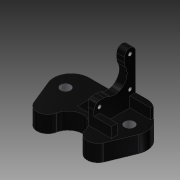
# Autodesk Inventor part: BackStopper
Saved by Autodesk Inventor 2015 (Build 190159000, 159)
## iProperties
Created: 2017-01-04
Part Number: BackStopper
Material: Generic
Document SubType Name: Modeling
Designer: Ernest
Density: 1 g/cm^3
Appearance: Default
Mass: 71.4554 g
Surface Area: 189.352 cm^2
Volume: 71.4554 cm^3
Author: Ernest
Autodesk Inventor part; units mm, degrees
ref_plane "YZ Plane" through (0, 0, 0) normal (1, 0, 0) x (0, 1, 0)
ref_plane "XZ Plane" through (0, 0, 0) normal (0, 1, 0) x (-1, 0, 0)
ref_plane "XY Plane" through (0, 0, 0) normal (0, 0, 1) x (1, 0, 0)
sketch "Sketch1" plane through (0, 0, 0) normal (0, 0, 1) x (1, 0, 0)
  circle A0 centre (0, 0) radius 8
  circle A1 centre (25.5147, 5) radius 3
  circle A2 centre (-25.5147, 5) radius 3
  circle A3 centre (32.5, 30) radius 5
  circle A4 centre (-32.5, 30) radius 5
  arc A5 (45.4578, 24.6994) -> (32.5, 44) centre (32.5, 30) ccw
  arc A6 (-32.5, 44) -> (-45.4578, 24.6994) centre (-32.5, 30) ccw
  line L0 (-24.3676, 0) -> (22.7562, 0) construction
  line L1 (-38.3266, 30) -> (45.5284, 30) construction
  line L2 (-33.7528, 8) -> (48.0284, 8) construction
  circle A7 centre (-25.5147, 5) radius 6
  circle A8 centre (25.5147, 5) radius 6
  arc A9 (14.72, 2.8846) -> (-15, 0) centre (0, 0) ccw
  arc A10 (-35.6958, 0.8353) -> (-14.72, 2.8846) centre (-25.5147, 5) ccw
  arc A11 (14.72, 2.8846) -> (35.6958, 0.8353) centre (25.5147, 5) ccw
  line L3 (-45.4578, 24.6994) -> (-35.6958, 0.8353)
  line L4 (35.6958, 0.8353) -> (45.4578, 24.6994)
  line L5 (-32.5, 44) -> (32.5, 44)
  dimension "d0" = 65
  dimension "d1" = 32.5
  dimension "d2" = 10
  dimension "d3" = 10
  dimension "d4" = 6
  dimension "d5" = 6
  dimension "d6" = 28
  dimension "d7" = 28
  dimension "d14" = 16
  dimension "d16" = 15
  dimension "d18" = 12
  dimension "d19" = 12
  dimension "d20" = 30
  dimension "d33" = 30
  dimension "d34" = 15
  constraints: 12 centre point, 12 end point, 11 point on circle, 10 tangent, 8 coincident, 4 horizontal, 4 point on line, 2 parallel
  measures "d0" distance of A3.centre A4.centre
  measures "d1" horizontal distance of point (0, 0) A4.centre
  measures "d2" diameter of A4
  measures "d3" diameter of A3
  measures "d4" diameter of A2
  measures "d5" diameter of A1
  measures "d6" diameter of A5
  measures "d7" diameter of A6
  measures "d14" diameter of A0
  measures "d18" diameter of A7
  measures "d19" diameter of A8
  measures "d20" diameter of A9
  measures "d33" distance from line of point (0, 0) L1
extrude "Extrusion1" add sketch "Sketch1" along normal blind 12 contours L4 A11 A9 A10 L3 A6 L5 A5 | A7 | A8
sketch "Sketch2" plane through (0, 0, 12) normal (0, 0, 1) x (1, 0, 0)
  circle A0 centre (25.5147, 5) radius 3 projected
  circle A1 centre (-25.5147, 5) radius 3 projected
  circle A2 centre (-32.5, 30) radius 5 projected
  circle A3 centre (32.5, 30) radius 5 projected
  line L0 (-45.4578, 24.6994) -> (-35.6958, 0.8353) projected
  arc A4 (-35.6958, 0.8353) -> (-14.72, 2.8846) centre (-25.5147, 5) ccw projected
  arc A5 (14.72, 2.8846) -> (-14.72, 2.8846) centre (0, 0) ccw projected
  arc A6 (14.72, 2.8846) -> (35.6958, 0.8353) centre (25.5147, 5) ccw projected
  line L1 (35.6958, 0.8353) -> (45.4578, 24.6994) projected
  arc A7 (45.4578, 24.6994) -> (32.5, 44) centre (32.5, 30) ccw projected
  line L2 (32.5, 44) -> (-32.5, 44) projected
  arc A8 (-32.5, 44) -> (-45.4578, 24.6994) centre (-32.5, 30) ccw projected
  circle A9 centre (-32.5, 30) radius 5 projected
  circle A10 centre (-32.5, 30) radius 7.5
  circle A11 centre (32.5, 30) radius 5
  constraints: 2 centre point, 2 coincident, 1 concentric
extrude "Extrusion2" add sketch "Sketch2" along normal blind 5 contours A0 | A1 | A8 L2 A7 L1 A6 A5 A4 L0 | A10
sketch "Sketch3" plane through (0, 0, 17) normal (0, 0, 1) x (1, 0, 0)
  line L0 (-10, 39.5) -> (10, 39.5)
  line L1 (10, 39.5) -> (10, 19.5)
  line L2 (10, 19.5) -> (-10, 19.5)
  line L3 (-10, 19.5) -> (-10, 39.5)
  circle A0 centre (32.5, 30) radius 5 projected
  circle A1 centre (-32.5, 30) radius 5 projected
  line L4 (-45.4578, 24.6994) -> (-35.6958, 0.8353) projected
  arc A2 (-35.6958, 0.8353) -> (-14.72, 2.8846) centre (-25.5147, 5) ccw projected
  arc A3 (14.72, 2.8846) -> (-14.72, 2.8846) centre (0, 0) ccw projected
  arc A4 (14.72, 2.8846) -> (35.6958, 0.8353) centre (25.5147, 5) ccw projected
  line L5 (35.6958, 0.8353) -> (45.4578, 24.6994) projected
  arc A5 (45.4578, 24.6994) -> (32.5, 44) centre (32.5, 30) ccw projected
  line L6 (32.5, 44) -> (-32.5, 44) projected
  arc A6 (-32.5, 44) -> (-45.4578, 24.6994) centre (-32.5, 30) ccw projected
  dimension "d25" = 20
  dimension "d26" = 20
  dimension "d27" = 10
  dimension "d29" = 4.5
  dimension "d32" = 29
  constraints: 8 end point, 2 parallel, 1 horizontal, 1 perpendicular
  measures "d25" distance between parallel lines of L2 L0
  measures "d26" distance between parallel lines of L1 L3
  measures "d27" distance from line of point (0, 0) L3
  measures "d29" distance between parallel lines of L6 L0
  measures "d32" distance edge to line of A3 L6
extrude "Extrusion3" cut sketch "Sketch3" against normal blind 17 contours L0 L1 L2 L3
sketch "Sketch7" plane through (0, 0, 17) normal (0, 0, 1) x (1, 0, 0)
  line L0 (-10, 19.5) -> (-10, 39.5) projected
  line L1 (-10, 39.5) -> (10, 39.5) projected
  line L2 (10, 39.5) -> (10, 19.5) projected
  line L3 (10, 19.5) -> (-10, 19.5) projected
  circle A0 centre (32.5, 30) radius 5 projected
  circle A1 centre (-32.5, 30) radius 5 projected
  line L4 (-45.4578, 24.6994) -> (-35.6958, 0.8353) projected
  arc A2 (-35.6958, 0.8353) -> (-14.72, 2.8846) centre (-25.5147, 5) ccw projected
  arc A3 (14.72, 2.8846) -> (-14.72, 2.8846) centre (0, 0) ccw projected
  arc A4 (14.72, 2.8846) -> (35.6958, 0.8353) centre (25.5147, 5) ccw projected
  line L5 (35.6958, 0.8353) -> (45.4578, 24.6994) projected
  arc A5 (45.4578, 24.6994) -> (32.5, 44) centre (32.5, 30) ccw projected
  line L6 (32.5, 44) -> (-32.5, 44) projected
  arc A6 (-32.5, 44) -> (-45.4578, 24.6994) centre (-32.5, 30) ccw projected
  line L7 (-32.5, 44) -> (32.5, 44)
  line L8 (32.5, 44) -> (32.5, 50.7)
  line L9 (29.2827, 50.7) -> (-29.2827, 50.7)
  line L10 (-32.5, 50.7) -> (-32.5, 44)
  line L11 (45.9427, 25.885) -> (35.6958, 0.8353)
  arc A7 (45.9427, 25.885) -> (29.2827, 50.7) centre (29.2827, 32.7) ccw
  line L12 (-45.9427, 25.885) -> (-35.6958, 0.8353)
  arc A8 (-29.2827, 50.7) -> (-45.9427, 25.885) centre (-29.2827, 32.7) ccw
  circle A9 centre (-32.5, 30) radius 5 projected
  arc A10 (-32.5, 44) -> (-45.4578, 24.6994) centre (-32.5, 30) ccw
  arc A11 (45.4578, 24.6994) -> (32.5, 44) centre (32.5, 30) ccw
  dimension "d55" = 6.7
  dimension "d56" = 18
  dimension "d57" = 18
  constraints: 12 end point, 8 point on circle, 4 centre point, 4 point on line, 4 tangent, 2 coincident, 2 concentric, 2 parallel, 1 collinear, 1 horizontal, 1 perpendicular
  measures "d55" distance of L8.end L7.end
  measures "d56" radius of A7
  measures "d57" radius of A8
extrude "Extrusion7" add sketch "Sketch7" against normal blind 17 contours L12 A8 L10 A6 | L10 A8 L9 A7 L8 L6 | L8 A7 L11 A5
sketch "Sketch8" plane through (0, 0, 17) normal (0, 0, 1) x (1, 0, 0)
  line L0 (-10, 19.5) -> (-10, 39.5) projected
  line L1 (-10, 39.5) -> (10, 39.5) projected
  line L2 (10, 39.5) -> (10, 19.5) projected
  line L3 (10, 19.5) -> (-10, 19.5) projected
  circle A0 centre (32.5, 30) radius 5 projected
  circle A1 centre (-32.5, 30) radius 5 projected
  line L4 (-45.9427, 25.885) -> (-35.6958, 0.8353) projected
  arc A2 (-35.6958, 0.8353) -> (-14.72, 2.8846) centre (-25.5147, 5) ccw projected
  arc A3 (14.72, 2.8846) -> (-14.72, 2.8846) centre (0, 0) ccw projected
  arc A4 (14.72, 2.8846) -> (35.6958, 0.8353) centre (25.5147, 5) ccw projected
  line L5 (35.6958, 0.8353) -> (45.9427, 25.885) projected
  arc A5 (45.9427, 25.885) -> (29.2827, 50.7) centre (29.2827, 32.7) ccw projected
  line L6 (29.2827, 50.7) -> (-29.2827, 50.7) projected
  arc A6 (-29.2827, 50.7) -> (-45.9427, 25.885) centre (-29.2827, 32.7) ccw projected
  line L7 (10, 50.7) -> (18, 50.7)
  line L8 (18, 50.7) -> (18, 8.4)
  line L9 (18, 8.4) -> (10, 8.4)
  line L10 (10, 8.4) -> (10, 50.7)
  line L11 (10, 39.5) -> (10, 19.5) projected
  line L12 (18, 50.7) -> (29.2827, 50.7)
  line L13 (29.2827, 50.7) -> (29.2827, 44.8229)
  line L14 (29.2827, 44.8229) -> (18, 44.8229)
  line L15 (18, 44.8229) -> (18, 50.7)
  line L16 (18, 8.4) -> (35.6958, 8.4)
  line L17 (35.6958, 8.4) -> (35.6958, 14.3153)
  line L18 (35.6958, 14.3153) -> (18, 14.3153)
  line L19 (18, 14.3153) -> (18, 8.4)
  line L20 (29.2827, 44.8229) -> (39.0827, 44.8229)
  line L21 (39.0827, 44.8229) -> (39.0827, 47.7984)
  arc A7 (39.0827, 47.7984) -> (29.2827, 50.7) centre (29.2827, 32.7) ccw
  dimension "d60" = 42.3
  dimension "d61" = 8
  constraints: 28 end point, 6 parallel, 4 horizontal, 4 perpendicular, 2 point on circle, 1 centre point, 1 coincident, 1 collinear, 1 concentric, 1 point on line
  measures "d60" distance of L7.end L8.end
  measures "d61" distance of L8.end L9.end
extrude "Extrusion8" add sketch "Sketch8" along normal blind 10.5 contours L2 L10 L6 L8 L9 A3 | A3 L9 L10 | L6 L13 L14 L8 | L8 L18 L17 L16 | A5 L21 L20 L13
sketch "Sketch9" plane through (10, 19.5, 0) normal (-1, 0, 0) x (0, 0, 1)
  line L0 (17, 20) -> (0, 20) projected
  line L1 (0, 0) -> (0, 20) projected
  line L2 (17, 0) -> (0, 0) projected
  line L3 (17, -8.3197) -> (17, 0) projected
  line L4 (17, -8.3197) -> (17, -11.1) projected
  line L5 (17, -11.1) -> (27.5, -11.1) projected
  line L6 (27.5, 31.2) -> (27.5, -11.1) projected
  line L7 (17, 31.2) -> (27.5, 31.2) projected
  line L8 (17, 20) -> (17, 31.2) projected
  arc A0 (54.5354, 21.0778) -> (37.6222, 4.1646) centre (48.65, 10.05) ccw
  circle A1 centre (33.15, 25.55) radius 1.75
  circle A2 centre (33.15, -5.45) radius 1.75
  circle A3 centre (64.15, 25.55) radius 1.75
  line L9 (27.5, 31.2) -> (69.8, 31.2)
  line L10 (59.2437, 19.9) -> (64.15, 19.9)
  arc A4 (64.15, 19.9) -> (64.15, 31.2) centre (64.15, 25.55) ccw
  arc A5 (33.15, -11.1) -> (38.8, -5.45) centre (33.15, -5.45) ccw
  line L11 (38.8, -5.45) -> (38.8, -0.5437)
  line L12 (27.5, -11.1) -> (33.15, -11.1)
  arc A6 (38.8, -0.5437) -> (37.6222, 4.1646) centre (28.8, -0.5437) ccw
  arc A7 (54.5354, 21.0778) -> (59.2437, 19.9) centre (59.2437, 29.9) ccw
  point P0 (0, -19.5)
  point P1 (56.3459, 19.9)
  point P2 (38.8, 2.3541)
  dimension "d64" = 25
  dimension "d65" = 21.15
  dimension "d66" = 21.15
  dimension "d67" = 5.65
  dimension "d68" = 5.65
  dimension "d69" = 5.65
  dimension "d70" = 5.65
  dimension "d71" = 5.65
  dimension "d72" = 31
  dimension "d73" = 3.5
  dimension "d74" = 3.5
  dimension "d75" = 3.5
  dimension "d76" = 42.3
  dimension "d77" = 5.65
  dimension "d78" = 11.3
  dimension "d79" = 10
  dimension "d80" = 10
  constraints: 12 point on circle, 8 centre point, 8 end point, 5 tangent, 3 point on line, 2 coincident, 2 horizontal, 1 vertical
  measures "d64" diameter of A0
  measures "d65" distance from line of L7 A0.centre
  measures "d66" distance from line of L6 A0.centre
  measures "d67" distance from line of L7 A1.centre
  measures "d68" distance from line of L6 A1.centre
  measures "d69" distance from line of L7 A3.centre
  measures "d70" distance from line of L6 A2.centre
  measures "d71" distance from line of L5 A2.centre
  measures "d72" distance of A1.centre A3.centre
  measures "d73" diameter of A1
  measures "d74" diameter of A3
  measures "d75" diameter of A2
  measures "d76" distance of L6.start L9.end
  measures "d77" distance from line of L10 A3.centre
  measures "d78" diameter of A5
  measures "d79" radius of A6
  measures "d80" radius of A7
extrude "Extrusion9" add sketch "Sketch9" against normal blind 8 contours L9 A4 L10 A7 A0 A6 L11 A5 L12 L6
sketch "Sketch10" plane through (0, 0, 17) normal (0, 0, -1) x (-1, 0, 0)
  arc A0 (-10, 11.1803) -> (-12.4274, 8.4) centre (0, 0) ccw
  line L0 (-12.4274, 8.4) -> (-10, 8.4)
  line L1 (-10, 8.4) -> (-10, 11.1803)
  constraints: 4 end point, 2 point on circle, 1 centre point, 1 coincident, 1 horizontal, 1 perpendicular
extrude "Extrusion10" cut sketch "Sketch10" against normal blind 41.25
equation "\"d1\" = 0.5 * d0"
equation "\"d27\" = 0.5 * d26"
equation "\"d29\" = 0.5 * d32 - 0.5 * d25"
body "Solid1"
